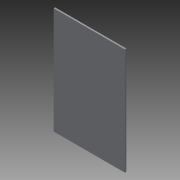
# Autodesk Inventor part: Part8
Saved by Autodesk Inventor 2015 (Build 190159000, 159)
## iProperties
Created: 2015-07-05
Part Number: Part8
Material: Generic
Document SubType Name: Modeling
Designer: tsayman
Density: 1 g/cm^3
Appearance: Default
Author: tsayman
Autodesk Inventor part; units mm, degrees
ref_plane "YZ Plane" through (0, 0, 0) normal (1, 0, 0) x (0, 1, 0)
ref_plane "XZ Plane" through (0, 0, 0) normal (0, 1, 0) x (-1, 0, 0)
ref_plane "XY Plane" through (0, 0, 0) normal (0, 0, 1) x (1, 0, 0)
sketch "Sketch1" plane through (0, 0, 0) normal (0, 0, 1) x (1, 0, 0)
  line L0 (-12.7, 712.819) -> (292.1, 712.819)
  line L1 (292.1, 712.819) -> (292.1, 255.619)
  line L2 (292.1, 255.619) -> (-12.7, 255.619)
  line L3 (-12.7, 255.619) -> (-12.7, 712.819)
  point P0 (0, 0)
  dimension "d0" = 304.8
  dimension "d1" = 457.2
  constraints: 8 end point, 2 parallel, 1 horizontal, 1 perpendicular
  measures "d0" distance of L1.end L2.end
  measures "d1" distance of L0.end L1.end
extrude "Extrusion1" add sketch "Sketch1" along normal blind 6.35
body "Solid1"
